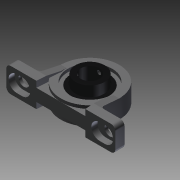
# Autodesk Inventor part: PBT12x
Saved by Autodesk Inventor 2011 SP1 (Build 150282100, 282)
## iProperties
Created: 2016-11-23
Part Number: PBT12x
Catalog Web Link: www.cadenas.de
Description: PBT, PBR, PBRS, PBRSX x-Ball Bearing Units - Pillow Type
Vendor: MISUMI
Document SubType Name: Modeling
Designer: psAdmin
Manufacturer: MISUMI
Mass: 15.1839 g
Surface Area: 74.2509 cm^2
Volume: 15.1839 cm^3
Density: 1 g/cm^3
Category: PARTsolutions
Company: MISUMI
Title: PBT12x
Author: Cadenas PARTsolutions
Comments: Ball Bearing Units - Pillow Type
PSOL_IDENT_0: {$CADENAS_DATA\23d-libs\misumi\metric\12_bearing_holders\pbt.prj},178 {VTYP=3D},{NB=PBT12x},{LINA=PB
PSOL_IDENT_1: T12x},{NN=PBT, PBR, PBRS, PBRSX x},{DATE=17.06.2016 05:47:22},{GEOMDATE=07.10.2008 07:41:00},{VERSIO
PSOL_IDENT_2: N=},{LINEID=190},{LINESUBID=-1},{WBVAR=TS,MAT}  {NB=PBT12x},{LINA=PBT12x},{KT=DUMMY},{PN=PBT12},{TYP
PSOL_IDENT_3: E=PBT},{TS=T},{MAT=},{MATH=Zinc Alloy Die Cast},{MATB=52100 Bearing Steel},{MATRS=Nitrile Rubber (NB
PSOL_IDENT_4: R)},{MATSS=4137 Alloy Steel},{MATER=-},{STER=-},{PRECISION=JIS B 1558/JIS B 1559},{OT=-10 ~+ 80},{D=
PSOL_IDENT_5: 12},{H=19},{L=71},{L1=56},{A=16},{DD=7},{TT=6},{TX1=6},{TX2=6},{H1=38.0},{H11=38},{H12=37.0},{B=14.5
PSOL_IDENT_6: },{B1=17.500},{B2=14.500},{S=4.0},{MASS=80},{CR=5100},{CR1=5100},{CR2=4300},{COR=2400},{COR1=2400},{
PSOL_IDENT_7: COR2=1900},{W1=80},{W2=91},{W3=98},{D1=19.000},{D2=12.000},{D3=38.000},{D4=40.000},{D5=29.000},{M1=M
PSOL_IDENT_8: 3 x 0.35},{M2=M4 x 0.7},{TT1=0.59},{TT2=1.5},{ALC1=0.35},{ALC2=0.88},{MMIN1=2.621},{MMIN2=3.242},{MM
PSOL_IDENT_9: AX1=3.000},{MMAX2=4.000},{M=M3 x 0.35},{T=0.59},{ALC=0.35},{MMIN=2.621},{MMAX=3},{MATALG=    '','Ste
PSOL_IDENT_10: el'     },{X=1},{DSCREW=3},{LSCREW=4},{DS1=3.000},{LS1=4.000},{DS2=4.000},{LS2=4.000}
NN: PBT, PBR, PBRS, PBRSX x
NT: Ball Bearing Units - Pillow Type
NB: PBT12x
NBSYN: $PN.x
LINA: PBT12x
PN: PBT12
TS: Set Screw
MAT: Steel
MATH: Zinc Alloy Die Cast
MATB: 52100 Bearing Steel
MATRS: Nitrile Rubber (NBR)
MATSS: 4137 Alloy Steel
MATER: -
PRECISION: JIS B 1558/JIS B 1559
OT: -10 ~+ 80
D: 12
H: 19
L: 71
L1: 56
A: 16
DD: 7
TT: 6
H1: 38.0
B: 14.5
S: 4.0
MASS: 80
CR: 5100
COR: 2400
M: M3 x 0.35
T: 0.59
ALC: 0.35
SUPPLIER: MISUMI
ARTICLENO: PBT12x
BOMINFO: PBT12x
CREATOR: CADENAS GmbH
Autodesk Inventor part; units mm, degrees
sketch "Sketch_1" plane through (0, 0, 0) normal (0, 0, 1) x (1, 0, 0)
  line L0 (-35.5, 0) -> (35.5, 0)
  line L1 (35.5, 0) -> (35.5, 6)
  line L2 (35.5, 6) -> (22.3241, 6)
  arc A0 (19.8307, 8.3179) -> (22.3241, 6) centre (22.3241, 8.5) ccw
  line L3 (19.8307, 8.3179) -> (18.9495, 20.3839)
  line L4 (18.9495, 20.3839) -> (15.162, 20.3839)
  arc A1 (-15.162, 20.3839) -> (15.162, 20.3839) centre (0, 19) ccw
  line L5 (-15.162, 20.3839) -> (-18.9495, 20.3839)
  line L6 (-18.9495, 20.3839) -> (-19.8307, 8.3179)
  arc A2 (-22.3241, 6) -> (-19.8307, 8.3179) centre (-22.3241, 8.5) ccw
  line L7 (-22.3241, 6) -> (-35.5, 6)
  line L8 (-35.5, 6) -> (-35.5, 0)
  constraints: 18 end point, 6 point on circle, 3 centre point
extrude "Extrusion1" add sketch "Sketch_1" along normal mid plane 16
sketch "Sketch_2" plane through (0, 0, 6) normal (0, 0, 1) x (1, 0, 0)
  line L0 (-15.9482, 0) -> (15.9482, 0)
  line L1 (15.9482, 0) -> (14.4867, 19)
  line L2 (14.4867, 19) -> (-14.4867, 19)
  line L3 (-14.4867, 19) -> (-15.9482, 0)
  constraints: 8 end point
extrude "Extrusion2" cut sketch "Sketch_2" along normal blind 8
sketch "Sketch_6" plane through (0, 0, -6) normal (0, 0, 1) x (1, 0, 0)
  line L0 (-15.9482, 0) -> (15.9482, 0)
  line L1 (15.9482, 0) -> (14.4867, 19)
  line L2 (14.4867, 19) -> (-14.4867, 19)
  line L3 (-14.4867, 19) -> (-15.9482, 0)
  constraints: 8 end point
extrude "Extrusion3" cut sketch "Sketch_6" against normal blind 8
sketch "Sketch_3" plane through (0, 0, 0) normal (1, 0, 0) x (0, 1, 0)
  line L0 (-19, 32) -> (-19, -32)
  line L1 (-19, -32) -> (57, -32)
  line L2 (57, -32) -> (57, 32)
  line L3 (57, 32) -> (-19, 32)
  line L4 (0, 8) -> (0, -8)
  line L5 (0, -8) -> (6, -8)
  line L6 (6, -8) -> (19, -6)
  line L7 (19, -6) -> (38, -6)
  line L8 (38, -6) -> (38, 6)
  line L9 (38, 6) -> (19, 6)
  line L10 (19, 6) -> (6, 8)
  line L11 (6, 8) -> (0, 8)
  constraints: 24 end point
extrude "Extrusion4" cut sketch "Sketch_3" along normal mid plane 71
sketch "Sketch_4" plane through (0, 0, 0) normal (0, 1, 0) x (-1, 0, 0)
  line L0 (142, 32) -> (-142, 32)
  line L1 (-142, 32) -> (-142, -32)
  line L2 (-142, -32) -> (142, -32)
  line L3 (142, -32) -> (142, 32)
  line L4 (35.5, -5.16) -> (35.5, 5.16)
  arc A0 (35.5, 5.16) -> (32.66, 8) centre (32.66, 5.16) ccw
  line L5 (32.66, 8) -> (-32.66, 8)
  arc A1 (-32.66, 8) -> (-35.5, 5.16) centre (-32.66, 5.16) ccw
  line L6 (-35.5, 5.16) -> (-35.5, -5.16)
  arc A2 (-35.5, -5.16) -> (-32.66, -8) centre (-32.66, -5.16) ccw
  line L7 (-32.66, -8) -> (32.66, -8)
  arc A3 (32.66, -8) -> (35.5, -5.16) centre (32.66, -5.16) ccw
  constraints: 16 end point, 8 point on circle, 4 centre point
extrude "Extrusion5" cut sketch "Sketch_4" along normal blind 6
sketch "Sketch_5" plane through (0, 0, 0) normal (1, 0, 0) x (0, 1, 0)
  line L0 (19, -4) -> (19, 10.5)
  line L1 (28.5, 10.5) -> (25, 10.5)
  line L2 (25, 10.5) -> (25, -4)
  line L3 (25, -4) -> (27.7833, -4)
  arc A0 (27.8833, -4) -> (27.7833, -4) centre (27.8333, -4) ccw
  line L4 (27.8833, -4) -> (31.275, -4)
  arc A1 (31.375, -4) -> (31.275, -4) centre (31.325, -4) ccw
  line L5 (31.375, -4) -> (33.5, -4)
  line L6 (33.5, -4) -> (33.5, -6)
  line L7 (33.5, -6) -> (38, -6)
  line L8 (38, -6) -> (38, 6)
  line L9 (38, 6) -> (33.5, 6)
  line L10 (33.5, 6) -> (33.5, 4)
  line L11 (33.5, 4) -> (31.375, 4)
  arc A2 (31.275, 4) -> (31.375, 4) centre (31.325, 4) ccw
  line L12 (31.275, 4) -> (29.1667, 4)
  line L13 (29.1667, 4) -> (29.1667, 3.3333)
  line L14 (29.1667, 3.3333) -> (27.8333, 3.3333)
  line L15 (27.8333, 3.3333) -> (27.8333, 4)
  line L16 (27.8333, 4) -> (28.5, 4)
  line L17 (28.5, 4) -> (28.5, 10.5)
  constraints: 36 end point, 6 point on circle, 3 centre point
revolve "Revolution1" add sketch "Sketch_5" angle 360 about axis through (0, 19, -4) along (0, 0, -1)
sketch "Sketch_7" plane through (0, 0, 4) normal (0, 0, 1) x (1, 0, 0)
  line L0 (-16.3329, -5) -> (16.3329, -5)
  line L1 (16.3329, -5) -> (15.3482, 7.8003)
  arc A0 (-15.3482, 7.8003) -> (15.3482, 7.8003) centre (0, 19) ccw
  line L2 (-15.3482, 7.8003) -> (-16.3329, -5)
  constraints: 6 end point, 2 point on circle, 1 centre point
extrude "Extrusion6" cut sketch "Sketch_7" along normal blind 8
sketch "Sketch_8" plane through (0, 0, -4) normal (0, 0, 1) x (1, 0, 0)
  line L0 (-16.3329, -5) -> (16.3329, -5)
  line L1 (16.3329, -5) -> (15.3482, 7.8003)
  arc A0 (-15.3482, 7.8003) -> (15.3482, 7.8003) centre (0, 19) ccw
  line L2 (-15.3482, 7.8003) -> (-16.3329, -5)
  constraints: 6 end point, 2 point on circle, 1 centre point
extrude "Extrusion7" cut sketch "Sketch_8" against normal blind 8
sketch "Sketch9" plane through (15.9482, 0, -8) normal (0, -1, 0) x (1, 0, 0)
  point P0 (-43.9482, 8)
hole "Hole1" at (-28, 0, 0) direction (0, 1, 0) diameter 7 depth 8
sketch "Sketch10" plane through (15.9482, 0, -8) normal (0, -1, 0) x (1, 0, 0)
  point P0 (12.0518, 8)
hole "Hole2" at (28, 0, 0) direction (0, 1, 0) diameter 7 depth 8
sketch "Sketch_13" plane through (0, 0, 0) normal (1, 0, 0) x (0, 1, 0)
  line L0 (24.5, 8.0938) -> (28.5, 8.0938)
  line L1 (28.5, 8.0938) -> (28.5, 6.5938)
  line L2 (28.5, 6.5938) -> (28.2295, 6.8643)
  line L3 (28.2295, 6.8643) -> (24.7705, 6.8643)
  line L4 (24.7705, 6.8643) -> (24.5, 6.5938)
  line L5 (24.5, 6.5938) -> (24.5, 8.0938)
  line L6 (24.5, 8.0938) -> (28.5, 8.0938)
  constraints: 14 end point
revolve "Revolution2" cut sketch "Sketch_13" angle 360 about axis through (0, 24.5, 8.0938) along (0, -1, 0)
thread "Thread1" size "M3x0.5" class "6H" standard "ISO Metric profile" length 3.459
sketch "Sketch_11" plane through (0, 0, 0) normal (0, 1, 0) x (-1, 0, 0)
  arc A0 (34.08, 0) -> (28.7467, 5.3333) centre (28.7467, 0) ccw
  line L0 (28.7467, 5.3333) -> (25.2133, 5.3333)
  arc A1 (25.2133, 5.3333) -> (19.88, 0) centre (25.2133, 0) ccw
  arc A2 (19.88, 0) -> (25.2133, -5.3333) centre (25.2133, 0) ccw
  line L1 (25.2133, -5.3333) -> (28.7467, -5.3333)
  arc A3 (28.7467, -5.3333) -> (34.08, 0) centre (28.7467, 0) ccw
  constraints: 8 point on circle, 4 centre point, 4 end point
sketch "Sketch_12" plane through (0, 0, 0) normal (0, 1, 0) x (-1, 0, 0)
  arc A0 (-19.88, 0) -> (-25.2133, 5.3333) centre (-25.2133, 0) ccw
  line L0 (-25.2133, 5.3333) -> (-28.7467, 5.3333)
  arc A1 (-28.7467, 5.3333) -> (-34.08, 0) centre (-28.7467, 0) ccw
  arc A2 (-34.08, 0) -> (-28.7467, -5.3333) centre (-28.7467, 0) ccw
  line L1 (-28.7467, -5.3333) -> (-25.2133, -5.3333)
  arc A3 (-25.2133, -5.3333) -> (-19.88, 0) centre (-25.2133, 0) ccw
  constraints: 8 point on circle, 4 centre point, 4 end point
extrude "Extrusion8" cut sketch "Sketch_11" along normal blind 4
extrude "Extrusion9" cut sketch "Sketch_12" along normal blind 4
sketch "Sketch_21" plane through (-5.1962, 16, 0) normal (0.5, -0.8660254, 0) x (-0.8660254, -0.5, 0)
  line L0 (3.5, -8.0938) -> (-0.5, -8.0938)
  line L1 (-0.5, -8.0938) -> (-0.5, -6.5938)
  line L2 (-0.5, -6.5938) -> (-0.2295, -6.8643)
  line L3 (-0.2295, -6.8643) -> (3.2295, -6.8643)
  line L4 (3.2295, -6.8643) -> (3.5, -6.5938)
  line L5 (3.5, -6.5938) -> (3.5, -8.0938)
  line L6 (3.5, -8.0938) -> (-0.5, -8.0938)
  constraints: 14 end point
revolve "Revolution3" cut sketch "Sketch_21" angle 360 about axis through (-8.2272, 14.25, 8.0938) along (-0.8660254, -0.5, 0)
thread "Thread2" size "M3x0.5" class "6H" standard "ISO Metric profile" length 3.459
ref_plane "to_screw_XY" through (0, 25, 8.0938) normal (0, 1, 0) x (1, 0, 0)
ref_plane "to_screw_YZ" through (0, 25, 8.0938) normal (1, 0, 0) x (0, 0, -1)
ref_plane "to_screw_ZX" through (0, 25, 8.0938) normal (0, 0, -1) x (0, 1, 0)
ref_plane "to_screw_s_XY" through (-5.1962, 16, 8.0938) normal (-0.8660254, -0.5, 0) x (0.5, -0.8660254, 0)
ref_plane "to_screw_s_YZ" through (-5.1962, 16, 8.0938) normal (0.5, -0.8660254, 0) x (0, 0, 1)
ref_plane "to_screw_s_ZX" through (-5.1962, 16, 8.0938) normal (0, 0, 1) x (-0.8660254, -0.5, 0)
body "Solid1"
